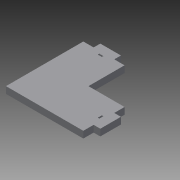
# Autodesk Inventor part: OVERHANG SUPPORT
Saved by Autodesk Inventor 2013 (Build 170138000, 138)
## iProperties
Created: 2014-03-04
Part Number: OVERHANG SUPPORT
Material: Generic
Document SubType Name: Modeling
Designer: employee
Density: 1 g/cm^3
Author: employee
Autodesk Inventor part; units mm, degrees
ref_plane "YZ Plane" through (0, 0, 0) normal (1, 0, 0) x (0, 1, 0)
ref_plane "XZ Plane" through (0, 0, 0) normal (0, 1, 0) x (-1, 0, 0)
ref_plane "XY Plane" through (0, 0, 0) normal (0, 0, 1) x (1, 0, 0)
sketch "Sketch1" plane through (0, 0, 0) normal (0, 0, 1) x (1, 0, 0)
  line L0 (0, 75) -> (0, 0)
  line L1 (0, 0) -> (75, 0)
  line L2 (75, 0) -> (75, 40)
  line L3 (75, 40) -> (40, 40)
  line L4 (40, 40) -> (40, 75)
  line L5 (40, 75) -> (0, 75)
  dimension "d0" = 75
  dimension "d2" = 40
  constraints: 12 end point, 4 parallel, 3 perpendicular, 1 vertical
  measures "d0" distance of L0.end L1.end
  measures "d2" distance of L1.end L2.end
extrude "Extrusion1" add sketch "Sketch1" along normal blind 6.477
sketch "Sketch2" plane through (0, 0, 6.477) normal (0, 0, 1) x (1, 0, 0)
  line L0 (75, 0) -> (75, 40) projected
  line L1 (40, 75) -> (0, 75) projected
  line L2 (10, 75) -> (30, 75)
  line L3 (30, 75) -> (30, 81.477)
  line L4 (30, 81.477) -> (10, 81.477)
  line L5 (10, 81.477) -> (10, 75)
  line L6 (75, 30) -> (81.477, 30)
  line L7 (81.477, 30) -> (81.477, 10)
  line L8 (81.477, 10) -> (75, 10)
  line L9 (75, 10) -> (75, 30)
  point P0 (75, 20)
  point P1 (20, 75)
  dimension "d5" = 6.477
  dimension "d7" = 20
  constraints: 16 end point, 4 midpoint, 4 parallel, 4 perpendicular, 2 horizontal, 2 point on line
  measures "d5" distance of L2.end L3.end
  measures "d7" distance of L3.end L4.end
extrude "Extrusion2" add sketch "Sketch2" against normal up to surface (6.477 mm away)
sketch "Sketch3" plane through (0, 0, 6.477) normal (0, 0, 1) x (1, 0, 0)
  line L0 (81.477, 10) -> (81.477, 30) projected
  line L1 (75, 30) -> (75, 40) projected
  line L2 (40, 75) -> (30, 75) projected
  line L3 (30, 81.477) -> (10, 81.477) projected
  line L4 (18, 72.5) -> (22, 72.5)
  line L5 (22, 72.5) -> (22, 71)
  line L6 (22, 71) -> (18, 71)
  line L7 (18, 71) -> (18, 72.5)
  line L8 (72.5, 18) -> (71, 18)
  line L9 (71, 18) -> (71, 22)
  line L10 (71, 22) -> (72.5, 22)
  line L11 (72.5, 22) -> (72.5, 18)
  point P0 (72.5, 20)
  point P1 (81.477, 20)
  point P2 (20, 72.5)
  point P3 (20, 81.477)
  dimension "d10" = 2.5
  dimension "d11" = 2.5
  dimension "d12" = 1.5
  dimension "d13" = 4
  constraints: 16 end point, 4 midpoint, 4 parallel, 4 perpendicular, 2 horizontal, 1 horizontal alignment, 1 vertical alignment
  measures "d10" distance between parallel lines of L2 L4
  measures "d11" distance between parallel lines of L1 L11
  measures "d12" distance of L4.end L5.end
  measures "d13" distance of L5.end L6.end
extrude "Extrusion3" cut sketch "Sketch3" against normal through all
body "Solid1"
